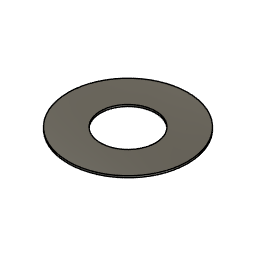
Cyclotron Base Plate v2 (Autodesk Fusion 360 design; units mm, degrees)
Autodesk Fusion 360 part; units mm, degrees
cylinder "CylinderPrimitive1" add diameter 165.1 height 2.3813 placed x (1, 0, 0) y (0, 1, 0) z (0, 0, 1) at (0, 0, 0)
hole "Hole1" at (0, 0, 2.3813) direction (0, 0, -1) diameter 76.2 depth 30.48 tip angle 118
equation "d1 = ( 1.5 / 16 ) * 1 in"
